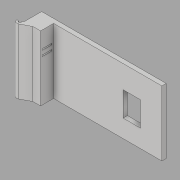
# Autodesk Inventor part: sliding servo release
Saved by Autodesk Inventor 2017 (Build 210142000, 142)
## iProperties
Created: 2019-05-09
Part Number: sliding servo release
Material: Generic
Document SubType Name: Modeling
Designer: Joe Sedutto
Density: 1 g/cm^3
Appearance: Default
Author: Joe Sedutto
Autodesk Inventor part; units mm, degrees
ref_plane "YZ Plane" through (0, 0, 0) normal (1, 0, 0) x (0, 1, 0)
ref_plane "XZ Plane" through (0, 0, 0) normal (0, 1, 0) x (-1, 0, 0)
ref_plane "XY Plane" through (0, 0, 0) normal (0, 0, 1) x (1, 0, 0)
sketch "Sketch1" plane through (0, 0, 0) normal (1, 0, 0) x (0, 1, 0)
  line L0 (0, 0) -> (76.2, 0)
  line L1 (76.2, 0) -> (76.2, -15.24)
  line L2 (76.2, -15.24) -> (0, -15.24)
  line L3 (0, -15.24) -> (0, 0)
  line L4 (57.15, -1.905) -> (55.5625, -1.905)
  line L5 (55.5625, -1.905) -> (55.5625, -13.335)
  line L6 (55.5625, -13.335) -> (57.15, -13.335)
  line L7 (57.15, -13.335) -> (57.15, -1.905)
  line L8 (50.8, -1.905) -> (49.2125, -1.905)
  line L9 (49.2125, -1.905) -> (49.2125, -13.335)
  line L10 (49.2125, -13.335) -> (50.8, -13.335)
  line L11 (50.8, -13.335) -> (50.8, -1.905)
  line L12 (57.15, -1.905) -> (57.15, 0) construction
  line L13 (57.15, -13.335) -> (57.15, -15.24) construction
  dimension "d0" = 76.2
  dimension "d1" = 15.24
  dimension "d2" = 4.7625
  dimension "d3" = 1.5875
  dimension "d4" = 19.05
  dimension "d5" = 11.43
  constraints: 28 end point, 6 parallel, 5 point on line, 3 horizontal, 3 perpendicular, 2 collinear, 1 vertical
  measures "d0" distance of L1.end L2.end
  measures "d1" distance of L0.end L1.end
  measures "d2" distance between parallel lines of L11 L5
  measures "d3" distance of L5.end L6.end
  measures "d4" distance between parallel lines of L1 L7
  measures "d5" distance between parallel lines of L6 L4
extrude "Extrusion1" add sketch "Sketch1" along normal blind 19.05
sketch "Sketch2" plane through (0, 0, -15.24) normal (0, 0, -1) x (-1, 0, 0)
  line L0 (0, 76.2) -> (0, 0) projected
  line L1 (0, 76.2) -> (-19.05, 76.2) projected
  line L2 (-19.05, 0) -> (-19.05, 76.2) projected
  line L3 (0, 0) -> (-19.05, 0) projected
  line L4 (0, 0) -> (0, 76.2) projected
  line L5 (0, 76.2) -> (-146.05, 76.2)
  line L6 (-146.05, 76.2) -> (-146.05, 0)
  line L7 (-146.05, 0) -> (0, 0)
  line L8 (0, 0) -> (0, 76.2)
  line L9 (0, 0) -> (-19.05, 0) projected
  line L10 (-120.9808, 49.6332) -> (-100.5958, 49.6332)
  line L11 (-100.5958, 49.6332) -> (-100.5958, 20.8282)
  line L12 (-100.5958, 20.8282) -> (-120.9808, 20.8282)
  line L13 (-120.9808, 20.8282) -> (-120.9808, 49.6332)
  dimension "d8" = 127
  constraints: 16 end point, 4 parallel, 2 horizontal, 2 perpendicular, 1 collinear
  measures "d8" distance between parallel lines of L2 L6
extrude "Extrusion2" add sketch "Sketch2" along normal blind 5.08
sketch "Sketch3" plane through (0, 76.2, 0) normal (0, 1, 0) x (1, 0, 0)
  arc A0 (-4.1469, -2.5594) -> (-1.4368, -1.4368) centre (-2.5594, -2.5594) ccw
  arc A1 (-6.1789, -2.5594) -> (0, 0) centre (-2.5594, -2.5594) ccw
  line L0 (-4.1469, -2.5594) -> (-6.1789, -2.5594)
  line L1 (0, 0) -> (19.05, 0) projected
  line L2 (-2.5594, -2.5594) -> (-4.1469, -2.5594) construction
  line L3 (0, 0) -> (-1.4368, -1.4368)
  line L4 (-2.5594, -2.5594) -> (-1.4368, -1.4368) construction
  line L5 (-0.8838, -5.7677) -> (10.16, 0)
  line L6 (0, 0) -> (0, 20.32) projected
  dimension "d11" = 3.175
  dimension "d12" = 2.032
  dimension "d14" = 135
  dimension "d15" = 10.16
  constraints: 11 end point, 5 point on circle, 2 centre point, 2 collinear, 1 horizontal, 1 point on line, 1 tangent
  measures "d11" diameter of A0
  measures "d12" radial gap between concentric circles of A0 A1
  measures "d14" angle of L1 L3
  measures "d15" distance from line of L5.end L6
extrude "Extrusion3" add sketch "Sketch3" against normal blind 76.2
body "Solid1"
